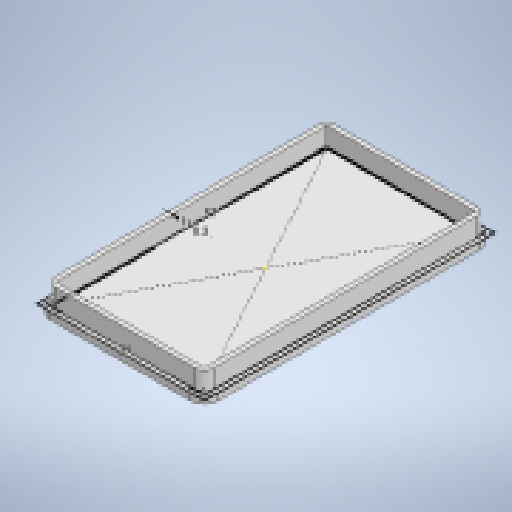
# Autodesk Inventor part: Part1
Saved by Autodesk Inventor 2025.2 (Build 292293000, 293)
## iProperties
Created: 2026-02-22
Part Number: Part1
Material: 一般
Document SubType Name: Modeling
Designer: naka6
Density: 1 g/cm^3
Appearance: 既定
Author: naka6
Autodesk Inventor part; units mm, degrees
ref_plane "YZ Plane" through (0, 0, 0) normal (1, 0, 0) x (0, 1, 0)
ref_plane "XZ Plane" through (0, 0, 0) normal (0, 1, 0) x (-1, 0, 0)
ref_plane "XY Plane" through (0, 0, 0) normal (0, 0, 1) x (1, 0, 0)
sketch "スケッチ1" plane through (0, 0, 0) normal (0, 1, 0) x (-1, 0, 0)
  line L0 (15.5, -28.5) -> (-15.5, -28.5)
  line L1 (-15.5, -28.5) -> (-15.5, 28.5)
  line L2 (-15.5, 28.5) -> (15.5, 28.5)
  line L3 (15.5, 28.5) -> (15.5, -28.5)
  line L4 (15.5, -28.5) -> (-15.5, 28.5) construction
  line L5 (-15.5, -28.5) -> (15.5, 28.5) construction
  line L6 (15.8, -28.8) -> (-15.8, -28.8)
  line L7 (-15.8, -28.8) -> (-15.8, 28.8)
  line L8 (-15.8, 28.8) -> (15.8, 28.8)
  line L9 (15.8, 28.8) -> (15.8, -28.8)
  line L10 (16.8, -29.8) -> (-16.8, -29.8)
  line L11 (-16.8, -29.8) -> (-16.8, 29.8)
  line L12 (-16.8, 29.8) -> (16.8, 29.8)
  line L13 (16.8, 29.8) -> (16.8, -29.8)
  line L14 (17.8, -30.8) -> (-17.8, -30.8)
  line L15 (-17.8, -30.8) -> (-17.8, 30.8)
  line L16 (-17.8, 30.8) -> (17.8, 30.8)
  line L17 (17.8, 30.8) -> (17.8, -30.8)
  point P0 (0, 0)
  dimension "d0" = 31
  dimension "d1" = 57
  dimension "d2" = 0.3
  dimension "d3" = 1
  dimension "d4" = 1
  constraints: 36 end point, 8 parallel, 4 perpendicular, 2 midpoint, 1 horizontal, 9 other
  measures "d0" distance of L1.end L2.end
  measures "d1" distance of L2.end L0.start
  measures "d2" distance between parallel lines of L3 L9
  measures "d3" distance between parallel lines of L9 L13
  measures "d4" distance between parallel lines of L13 L17
extrude "押し出し1" add sketch "スケッチ1" against normal blind 1.5 contours L0 L1 L2 L3 | L6 L7 L8 L9 | L10 L11 L12 L13 | L14 L15 L16 L17
extrude "押し出し2" add sketch "スケッチ1" along normal blind 4 contours L10 L11 L12 L13
fillet "フィレット1" radius 2 4 edges at (16.8, 2, 29.8) (16.8, 2, -29.8) (-16.8, 2, -29.8) (-16.8, 2, 29.8)
fillet "フィレット2" radius 3 4 edges at (-17.8, -0.75, 30.8) (-17.8, -0.75, -30.8) (17.8, -0.75, 30.8) (17.8, -0.75, -30.8)
sketch "スケッチ2" plane through (0, 0, 0) normal (0, 1, 0) x (1, 0, 0)
  point P0 (0, 0)
